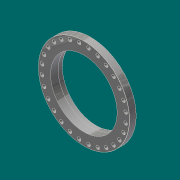
# Autodesk Inventor part: A1-19027-300-03 32in CL150 FFWN flange
Saved by Autodesk Inventor 2017.3 (Build 213257000, 257)
## iProperties
Created: 2011-05-31
Part Number: A1-19027-300-03 32in CL150 FFWN flange
Document SubType Name: Modeling
Designer: Graeme_Van_Dongen
Density: 7.85 g/cm^3
Description: 32" x 3/4" WALL CLASS 150 FFWN FLANGE, A105N
Material: A105N
Mass: 243295 g
Surface Area: 17304.5 cm^2
Volume: 30993 cm^3
Appearance: Steel
Author: Graeme_Van_Dongen
Autodesk Inventor part; units mm, degrees
ref_plane "YZ Plane" through (0, 0, 0) normal (1, 0, 0) x (0, 1, 0)
ref_plane "XZ Plane" through (0, 0, 0) normal (0, 1, 0) x (-1, 0, 0)
ref_plane "XY Plane" through (0, 0, 0) normal (0, 0, 1) x (1, 0, 0)
sketch "Sketch1" plane through (0, 0, 0) normal (0, 0, 1) x (1, 0, 0)
  circle A0 centre (0, 0) radius 530.225
  circle A1 centre (0, 0) radius 393.7
  dimension "d0" = 1060.45
  dimension "d1" = 787.4
  constraints: 2 centre point, 2 coincident
  measures "d0" diameter of A0
  measures "d1" diameter of A1
extrude "Extrusion1" add sketch "Sketch1" along normal blind 79.375
sketch "Sketch2" plane through (0, 0, 79.375) normal (0, 0, 1) x (1, 0, 0)
  circle A0 centre (0, 0) radius 393.7 projected
  circle A1 centre (0, 0) radius 530.225 projected
  circle A2 centre (0, 0) radius 457.2
  dimension "d4" = 914.4
  constraints: 1 centre point, 1 coincident
  measures "d4" diameter of A2
extrude "Extrusion2" add sketch "Sketch2" along normal blind 1.5875 contours A2
sketch "Sketch3" plane through (0, 0, 0) normal (0, 0, -1) x (-1, 0, 0)
  circle A0 centre (0, 0) radius 393.7 projected
  circle A1 centre (0, 0) radius 530.225 projected
  circle A2 centre (0, 0) radius 415.925
  dimension "d7" = 831.85
  constraints: 1 centre point, 1 coincident
  measures "d7" diameter of A2
extrude "Extrusion3" add sketch "Sketch3" along normal blind 63.5 contours A2
sketch "Sketch4" plane through (0, 0, 80.9625) normal (0, 0, 1) x (1, 0, 0)
  circle A0 centre (0, 0) radius 457.2 projected
  line L0 (0, -742.315) -> (0, 742.315) projected
  line L1 (-742.315, 0) -> (742.315, 0) projected
  line L2 (0, 0) -> (54.745, 485.8756) construction
  dimension "d13" = 488.95
  dimension "d14" = 6.429
  constraints: 2 end point
  measures "d13" distance of L2.start L2.end
  measures "d14" angle of L0 L2
hole "Hole1" at (54.745, 485.8756, 80.9625) direction (0, 0, -1) diameter 41.275 end through all
chamfer "Chamfer3" distance 0.7937 angle 45 2 edges at (54.745, 506.5131, 0) (54.745, 506.5131, 79.375)
pattern_circular "Circular Pattern1" count 28 over 360 about axis through (0, 0, -10) along (0, 0, -1) of "Hole1", "Chamfer3"
chamfer "Chamfer2" distance 1.5875 angle 45 2 edges at (-530.225, 0, 79.375) (-530.225, 0, 0)
fillet "Fillet2" radius 11.1125 1 edges at (415.925, 0, 0)
sketch "Sketch9" plane through (0, 0, 0) normal (1, 0, 0) x (0, 1, 0)
  line L0 (415.925, -11.1125) -> (415.925, -63.5) projected
  arc A0 (427.0375, 0) -> (415.925, -11.1125) centre (427.0375, -11.1125) ccw construction
  arc A1 (416.5952, -7.3118) -> (415.925, -11.1125) centre (427.0375, -11.1125) ccw
  line L1 (416.5952, -7.3118) -> (407.1659, -33.2185)
  line L2 (395.2875, -63.5) -> (415.925, -63.5)
  line L3 (406.4, -54.9731) -> (406.4, -37.5621)
  arc A2 (407.1659, -33.2185) -> (406.4, -37.5621) centre (419.1, -37.5621) ccw
  line L4 (0, -87.3125) -> (0, 112.7125) projected
  line L5 (393.7, -63.5) -> (393.7, 80.9625) construction
  line L6 (406.4, -54.9731) -> (395.2875, -63.5)
  point P0 (0, 0)
  dimension "d77" = 20
  dimension "d78" = 406.4
  dimension "d79" = 12.7
  dimension "d84" = 37.5
  dimension "d85" = 11.1125
  constraints: 9 end point, 5 point on circle, 3 tangent, 2 centre point, 1 concentric, 1 point on line, 1 vertical
  measures "d77" angle of L0 L1
  measures "d78" distance from line of point (0, 0) L3
  measures "d79" radius of A2
  measures "d84" angle of L2 L6
  measures "d85" horizontal distance of L3.start L2.start
revolve "Revolution3" cut sketch "Sketch9" angle 360 about axis through (0, 0, -10) along (0, 0, 1)
sketch "Sketch13" plane through (0, 0, 80.9625) normal (0, 0, 1) x (1, 0, 0)
  circle A0 centre (0, 0) radius 393.7 projected
  circle A1 centre (0, 0) radius 457.2 projected
extrude "Extrusion6" cut sketch "Sketch13" against normal blind 1.5875
sketch "Sketch14" plane through (0, 0, 79.375) normal (0, 0, 1) x (1, 0, 0)
  circle A0 centre (0, 0) radius 387.35
  circle A1 centre (0, 0) radius 393.7 projected
  dimension "d121" = 774.7
  constraints: 1 centre point, 1 coincident
  measures "d121" diameter of A0
extrude "Extrusion7" add sketch "Sketch14" against normal blind 88.9
fillet "Fillet5" radius 0.7937 1 edges at (393.7, 0, -9.525)
chamfer "Chamfer9" distance 0.7937 angle 45 1 edges at (-387.35, 0, -9.525)
equation "\"d0\" = OD"
equation "\"d1\" = Bore"
equation "\"d2\" = Thickness"
equation "\"d4\" = RFDia"
equation "\"d5\" = RFDepth"
equation "\"d7\" = NeckDia"
equation "\"d8\" = NeckLength"
equation "\"d13\" = 0.5 * BCD"
equation "\"d15\" = HoleDia"
equation "\"d30\" = HoleChamfer"
equation "\"d25\" = RimChamfer"
equation "\"d29\" = NeckFillet"
equation "\"OD\" = 1060.45"
equation "\"Bore\" = 787.4"
equation "\"Thickness\" = 79.375"
equation "\"RFDia\" = 914.4"
equation "\"RFDepth\" = 1.5875"
equation "\"HoleDia\" = 41.275"
equation "\"BCD\" = 977.9"
equation "\"NeckDia\" = 831.85"
equation "\"NeckLength\" = 63.5"
equation "\"HoleChamfer\" = 0.79375"
equation "\"RimChamfer\" = 1.5875"
equation "\"NeckChamfer\" = 1.5875"
equation "\"NeckFillet\" = 11.1125"
body "Solid1"
